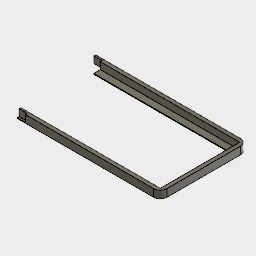
FrontFrame (Autodesk Fusion 360 design; units mm, degrees)
Autodesk Fusion 360 part; units mm, degrees
sketch "Skizze1" plane through (0, 0, 0) normal (0, 1, 0) x (1, 0, 0)
  line L0 (84, -47.75) -> (-84, -47.75)
  line L1 (-84, -47.75) -> (-84, 47.75)
  line L2 (-84, 47.75) -> (84, 47.75)
  line L3 (84, 47.75) -> (84, -47.75)
  line L4 (84, -47.75) -> (-84, 47.75) construction
  line L5 (-84, -47.75) -> (84, 47.75) construction
  line L6 (86.25, -50) -> (-86.25, -50)
  line L7 (-86.25, -50) -> (-86.25, 50)
  line L8 (-86.25, 50) -> (86.25, 50)
  line L9 (86.25, 50) -> (86.25, -50)
  line L10 (86.25, -50) -> (-86.25, 50) construction
  line L11 (-86.25, -50) -> (86.25, 50) construction
  line L12 (-84, 47.75) -> (-86.25, 47.75)
  line L13 (-84, -47.75) -> (-86.25, -47.75)
extrude "Extrusion1" add sketch "Skizze1" along normal blind 10 contours L0 L2 L3 L6 L7 L8 L9 L12 L13
sketch "Skizze2" plane through (0, 0, 0) normal (0, -1, 0) x (1, 0, 0)
  line L0 (84, -47.75) -> (-86.25, -47.75)
  line L1 (-86.25, -47.75) -> (-86.25, -50)
  line L2 (-86.25, -50) -> (86.25, -50)
  line L3 (86.25, -50) -> (86.25, 50)
  line L4 (86.25, 50) -> (-86.25, 50)
  line L5 (-86.25, 50) -> (-86.25, 47.75)
  line L6 (-86.25, 47.75) -> (84, 47.75)
  line L7 (84, 47.75) -> (84, -47.75)
  line L8 (-86.25, -47.75) -> (-86.25, -39.75)
  line L9 (84, 47.75) -> (84, 39.75)
  line L10 (84, 39.75) -> (76, 39.75)
  line L11 (76, 39.75) -> (-86.25, 39.75)
  line L12 (-86.25, 39.75) -> (-86.25, -39.75)
  line L13 (-86.25, -39.75) -> (76, -39.75)
  line L14 (76, -39.75) -> (76, 39.75)
  line L15 (-86.25, 47.75) -> (-86.25, 39.75)
extrude "Extrusion2" add sketch "Skizze2" against normal blind 1 contours L0 L7 L8 L10 L13 L14 | L6 L7 L9 L10 L11 L15
extrude "Extrusion3" add 1 faces at (28, 10, 49.25) along direction (0, 1, 0) blind 1
extrude "Extrusion4" add 1 faces at (28, 11, 49.25) along direction (0, 1, 0) blind 0.18
sketch "Skizze3" plane through (-86.25, 0, 0) normal (-1, 0, 0) x (0, 0, 1)
  line L0 (39.75, 0) -> (50, 0)
  line L1 (50, 0) -> (50, 11.18)
  line L2 (50, 11.18) -> (47.75, 11.18)
  line L3 (47.75, 11.18) -> (47.75, 1)
  line L4 (47.75, 1) -> (39.75, 1)
  line L5 (39.75, 1) -> (39.75, 0)
  line L6 (47.75, 1) -> (47.75, 0)
  line L7 (-39.75, 0) -> (-50, 0)
  line L8 (-50, 0) -> (50, 0)
  line L9 (-47.75, 1) -> (-47.75, 0)
  point P0 (-47.75, 1)
extrude "Extrusion5" cut sketch "Skizze3" against normal blind 20 contours L0 L1 L2 L3 L6 L8
sketch "Skizze4" plane through (-86.25, 0, 0) normal (-1, 0, 0) x (0, 0, 1)
  line L0 (-50, 0) -> (-39.75, 0)
  line L1 (-39.75, 0) -> (-39.75, 1)
  line L2 (-39.75, 1) -> (-47.75, 1)
  line L3 (-47.75, 1) -> (-47.75, 11.18)
  line L4 (-47.75, 11.18) -> (-50, 11.18)
  line L5 (-50, 11.18) -> (-50, 0)
  line L6 (-47.75, 1) -> (-47.75, 0)
extrude "Extrusion6" add sketch "Skizze4" along normal blind 20 contours L0 L3 L4 L5 L6
extrude "Extrusion7" add 1 faces at (-15.4167, 7.4533, 50) along direction (0, 0, 1) blind 2.25
extrude "Extrusion8" add 1 faces at (86.25, 3.7267, -15.9167) along direction (1, 0, 0) blind 2.25
extrude "Extrusion9" add 1 faces at (-41.3333, 3.7267, -50) along direction (0, 0, -1) blind 2.25
fillet "Abrundung1" radius 8 1 edges at (88.5, 5.59, 52.25)
fillet "Abrundung2" radius 8 1 edges at (88.5, 5.59, -52.25)
move_face "Flächen versetzen1" offset -2.5 1 faces at (-106.25, 4.06, -50.75)
extrude "Extrusion10" cut 1 faces at (-86.25, 0.3333, -45.0833) along direction (1, 0, 0) blind 2.5
extrude "Extrusion11" cut 1 faces at (-86.25, 0.3333, 45.0833) along direction (1, 0, 0) blind 2.5
extrude "Extrusion12" cut 1 faces at (-66.25, 4.06, 50.75) along direction (1, 0, 0) blind 2.5
sketch "Skizze5" plane through (0, 0, 0) normal (1, 0, 0) x (0, 0, -1)
extrude "Extrusion13" cut 1 faces at (-103.75, 4.06, -50.75) along direction (1, 0, 0) blind 20
extrude "Extrusion14" add 1 faces at (-63.75, 4.06, 50.75) along direction (-1, 0, 0) blind 20
sketch "Skizze6" plane through (-83.75, 0, 0) normal (-1, 0, 0) x (0, 0, 1)
  line L0 (47.75, 1) -> (39.75, 1)
  line L1 (39.75, 1) -> (39.75, 0)
  line L2 (39.75, 0) -> (52.25, 0)
  line L3 (52.25, 0) -> (52.25, 11.18)
  line L4 (52.25, 11.18) -> (47.75, 11.18)
  line L5 (47.75, 11.18) -> (47.75, 1)
  line L6 (47.75, 1) -> (52.25, 1)
extrude "Extrusion15" cut sketch "Skizze6" against normal blind 20 contours L3 L4 L5 L6
sketch "Skizze7" plane through (-83.75, 0, 0) normal (-1, 0, 0) x (0, 0, 1)
  line L0 (-52.25, 0) -> (-39.75, 0)
  line L1 (-39.75, 0) -> (-39.75, 1)
  line L2 (-39.75, 1) -> (-47.75, 1)
  line L3 (-47.75, 1) -> (-47.75, 11.18)
  line L4 (-47.75, 11.18) -> (-52.25, 11.18)
  line L5 (-52.25, 11.18) -> (-52.25, 0)
  line L6 (-47.75, 1) -> (-52.25, 1.0038)
extrude "Extrusion16" add sketch "Skizze7" along normal blind 20 contours L3 L4 L5 L6
extrude "Extrusion17" cut 1 faces at (-103.75, 4.3946, -49.25) along direction (1, 0, 0) blind 10
extrude "Extrusion18" add 1 faces at (-63.75, 4.3933, 49.25) along direction (-1, 0, 0) blind 10
sketch "Skizze8" plane through (-73.75, 0, 0) normal (-1, 0, 0) x (0, 0, 1)
  line L0 (47.75, 1) -> (52.25, 1)
  line L1 (52.25, 1) -> (52.25, 11.18)
  line L2 (52.25, 11.18) -> (47.75, 11.18)
  line L3 (47.75, 11.18) -> (47.75, 1)
  line L4 (50, 1) -> (50, 11.18)
extrude "Extrusion19" add sketch "Skizze8" along normal blind 10 contours L0 L2 L3 L4
sketch "Skizze9" plane through (-93.75, 0, 0) normal (-1, 0, 0) x (0, 0, 1)
  line L0 (-47.75, 11.18) -> (-52.25, 11.18)
  line L1 (-52.25, 11.18) -> (-52.25, 1.0038)
  line L2 (-52.25, 1.0038) -> (-47.75, 1)
  line L3 (-47.75, 1) -> (-47.75, 11.18)
  line L4 (-50, 11.18) -> (-50, 1.0019)
extrude "Extrusion20" cut sketch "Skizze9" against normal blind 10 contours L0 L2 L3 L4
extrude "Extrusion21" cut 1 faces at (26.9167, 11.18, -49.25) along direction (0, -1, 0) blind 2
